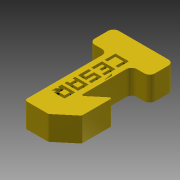
# Autodesk Inventor part: Part1
Saved by Autodesk Inventor 2014 (Build 180170000, 170)
## iProperties
Created: 2015-08-08
Part Number: Part1
Material: Generic
Document SubType Name: Modeling
Designer: Rubén
Density: 1 g/cm^3
Appearance: Glossy - Gold
Author: Rubén
Autodesk Inventor part; units mm, degrees
ref_plane "YZ Plane" through (0, 0, 0) normal (1, 0, 0) x (0, 1, 0)
ref_plane "XZ Plane" through (0, 0, 0) normal (0, 1, 0) x (-1, 0, 0)
ref_plane "XY Plane" through (0, 0, 0) normal (0, 0, 1) x (1, 0, 0)
sketch "Sketch1" plane through (0, 0, 0) normal (0, 1, 0) x (-1, 0, 0)
  line L0 (0, 0) -> (0, 38.5027)
  line L1 (0, 38.5027) -> (-13.5, 27.1748)
  line L2 (-13.5, 27.1748) -> (-13.5, 50.6722)
  line L3 (-13.5, 50.6722) -> (0, 62)
  line L4 (0, 62) -> (18, 62)
  line L5 (18, 62) -> (18, 0)
  line L6 (18, 0) -> (31.5, 0)
  line L7 (31.5, 0) -> (31.5, -18)
  line L8 (31.5, -18) -> (-13.5, -18)
  line L9 (-13.5, -18) -> (-13.5, 0)
  line L10 (-13.5, 0) -> (0, 0)
  dimension "d0" = 50
  dimension "d1" = 80
  dimension "d2" = 18
  dimension "d3" = 18
  dimension "d4" = 13.5
  dimension "d5" = 13.5
  dimension "d6" = 18
  dimension "d7" = 0
  dimension "d8" = 0
  dimension "d9" = 0
  constraints: 22 end point, 8 parallel, 1 perpendicular, 1 vertical
  measures "d0" angle of L1 L0
  measures "d1" distance between parallel lines of L8 L4
  measures "d2" distance between parallel lines of L5 L0
  measures "d3" distance of L8.end L9.end
  measures "d4" distance between parallel lines of L0 L9
  measures "d5" distance between parallel lines of L7 L5
  measures "d6" distance between parallel lines of L1 L3
  measures "d7" horizontal distance of L0.end L3.end
  measures "d8" distance between parallel lines of L9 L2
  measures "d9" vertical distance of L0.start L5.end
extrude "Extrusion1" add sketch "Sketch1" along normal blind 18
fillet "Fillet1" radius 2 3 edges at (-18, 9, 62) (0, 9, 62) (13.5, 9, 50.6722)
fillet "Fillet2" radius 1 2 edges at (0, 9, 38.5027) (13.5, 9, 27.1748)
fillet "Fillet3" radius 4 6 edges at (13.5, 9, 0) (13.5, 9, -18) (-31.5, 9, -18) (-18, 9, 0) (-31.5, 9, 0) (0, 9, 0)
sketch "Sketch2" plane through (0, 18, 0) normal (0, 1, 0) x (1, 0, 0)
  line L0 (-16, -62) -> (-0.7279, -62) projected
  line L1 (-4, 2) -> (-14, 2)
  line L2 (-14, -6) -> (-14, 2)
  line L3 (-4, 2) -> (-4, -6)
  line L4 (-4, -6) -> (-6, -6)
  line L5 (-6, -6) -> (-6, 0)
  line L6 (-6, 0) -> (-12, 0)
  line L7 (-12, 0) -> (-12, -6)
  line L8 (-12, -6) -> (-14, -6)
  line L9 (-4, -8) -> (-14, -8)
  line L10 (-14, -8) -> (-14, -16)
  line L11 (-12, -16) -> (-14, -16)
  line L12 (-12, -16) -> (-12, -10)
  line L13 (-12, -10) -> (-10, -10)
  line L14 (-10, -10) -> (-10, -14)
  line L15 (-10, -14) -> (-8, -14)
  line L16 (-8, -14) -> (-8, -10)
  line L17 (-8, -10) -> (-6, -10)
  line L18 (-6, -10) -> (-6, -16)
  line L19 (-6, -16) -> (-4, -16)
  line L20 (-4, -8) -> (-4, -16)
  line L21 (-4, -18) -> (-10, -18)
  line L22 (-10, -18) -> (-10, -24)
  line L23 (-10, -24) -> (-12, -24)
  line L24 (-12, -24) -> (-12, -18)
  line L25 (-12, -18) -> (-14, -18)
  line L26 (-14, -18) -> (-14, -26)
  line L27 (-14, -26) -> (-8, -26)
  line L28 (-8, -26) -> (-8, -20)
  line L29 (-8, -20) -> (-6, -20)
  line L30 (-6, -20) -> (-6, -26)
  line L31 (-6, -26) -> (-4, -26)
  line L32 (-4, -18) -> (-4, -26)
  line L33 (-4, -28) -> (-14, -28)
  line L34 (-14, -36) -> (-4, -36)
  line L35 (-4, -36) -> (-4, -28)
  line L36 (-6, -30) -> (-10, -30)
  line L37 (-10, -30) -> (-10, -34)
  line L38 (-4, -38) -> (-14, -38)
  line L39 (-1, -19.7264) -> (-2.5, -12)
  line L40 (-4, -6) -> (-4, -8) construction
  line L41 (-4, -16) -> (-4, -18) construction
  line L42 (-4, -26) -> (-4, -28) construction
  line L43 (-4, -36) -> (-4, -38) construction
  line L44 (-14, -36) -> (-14, -38) construction
  line L45 (-14, -6) -> (-14, -8) construction
  line L46 (-14, -26) -> (-14, -28) construction
  line L47 (-6, -26) -> (-8, -26) construction
  line L48 (-10, -18) -> (-12, -18) construction
  line L49 (-8, -20) -> (-8, -18) construction
  line L50 (-10, -24) -> (-8, -24) construction
  line L51 (-10, -24) -> (-10, -26) construction
  line L52 (-6, -10) -> (-6, -8) construction
  line L53 (-12, -30) -> (-14, -30)
  line L54 (-14, -30) -> (-14, -28)
  line L55 (-14, -34) -> (-14, -36)
  line L56 (-6, -30) -> (-6, -28) construction
  line L57 (-6, -30) -> (-6, -34)
  line L58 (-6, -34) -> (-6, -36) construction
  line L59 (-6, -30) -> (-4, -30) construction
  line L60 (-12, -30) -> (-12, -34)
  line L61 (-12, -34) -> (-14, -34)
  line L62 (-10, -30) -> (-12, -30) construction
  line L63 (-4, -38) -> (-4, -46)
  line L64 (-6, -40) -> (-6, -38) construction
  line L65 (-6, -40) -> (-4, -40) construction
  line L66 (-14, -38) -> (-14, -41)
  line L67 (-14, -41) -> (-12, -41)
  line L68 (-12, -41) -> (-14, -43)
  line L69 (-14, -43) -> (-14, -46)
  line L70 (-14, -46) -> (-12, -44)
  line L71 (-12, -44) -> (-12, -46)
  line L72 (-12, -46) -> (-4, -46)
  line L73 (-10, -40) -> (-10, -44)
  line L74 (-10, -44) -> (-6, -44)
  line L75 (-6, -44) -> (-6, -40)
  line L76 (-2.5, -12) -> (-1, -13.7264)
  line L77 (-12, -46) -> (-14, -46) construction
  line L78 (-14, -41) -> (-14, -43) construction
  line L79 (-6, -40) -> (-10, -40)
  line L80 (-10, -44) -> (-12, -44) construction
  line L81 (-14, -16) -> (-14, -18) construction
  line L82 (-6, -34) -> (-10, -34)
  line L83 (-1, -13.7264) -> (-1, -19.7264)
  line L84 (-1, -13.7264) -> (-1, -12) construction
  line L85 (-1, -12) -> (-2.5, -12) construction
  line L86 (-2.5, -12) -> (-4, -12) construction
  line L87 (-18, -4) -> (-18, -60) projected
  line L88 (0, -36.3582) -> (0, -4) projected
  line L89 (9.5, 18) -> (-27.5, 18) projected
  line L90 (-9, -46) -> (-9, -62) construction
  line L91 (-9, 2) -> (-9, 18) construction
  line L92 (-4, -22) -> (0, -22) construction
  line L93 (-14, -22) -> (-18, -22) construction
  point P0 (0, 0)
  dimension "d18" = 10
  dimension "d19" = 8
  dimension "d20" = 2
  dimension "d21" = 45
  dimension "d26" = 0
  dimension "d29" = 3
  dimension "d31" = 30
  constraints: 180 end point, 44 equal length, 41 perpendicular, 24 parallel, 20 collinear, 14 point on line, 5 midpoint
  measures "d18" distance of L1.start L1.end
  measures "d19" distance of L1.start L3.end
  measures "d20" distance between parallel lines of L19 L15
  measures "d21" angle of L67 L68
  measures "d26" distance from line of L71 L67.end
  measures "d29" distance between parallel lines of L20 L83
  measures "d31" angle of L39 L76
extrude "Extrusion2" cut sketch "Sketch2" against normal blind 3
body "Solid1"
